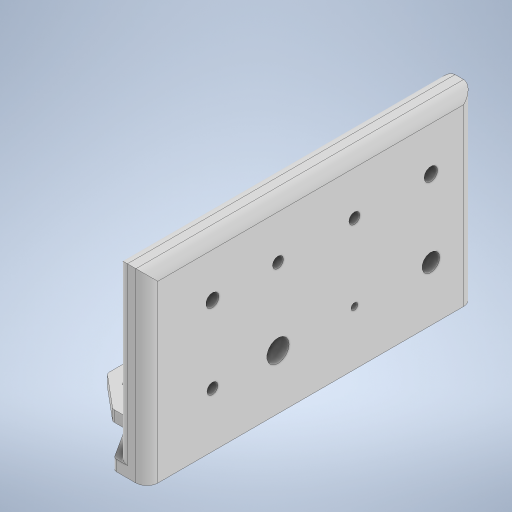
# Autodesk Inventor part: soporte_destornillador
Saved by Autodesk Inventor 2024 (Build 280153000, 153)
## iProperties
Created: 2023-06-27
Part Number: soporte_destornillador
Material: Generic
Document SubType Name: Modeling
Designer: LabTel_Admin
Density: 1 g/cm^3
Appearance: Default
Author: LabTel_Admin
Autodesk Inventor part; units mm, degrees
ref_plane "YZ Plane" through (0, 0, 0) normal (1, 0, 0) x (0, 1, 0)
ref_plane "XZ Plane" through (0, 0, 0) normal (0, 1, 0) x (-1, 0, 0)
ref_plane "XY Plane" through (0, 0, 0) normal (0, 0, 1) x (1, 0, 0)
sketch "Sketch2" plane through (0, 0, 0) normal (0, 1, 0) x (-1, 0, 0)
  line L0 (15.1065, 40) -> (17.4159, 44)
  line L1 (17.4159, 44) -> (22.0347, 44)
  line L2 (22.0347, 44) -> (24.3441, 40)
  line L3 (24.3441, 40) -> (22.0347, 36)
  line L4 (22.0347, 36) -> (17.4159, 36)
  line L5 (17.4159, 36) -> (15.1065, 40)
  circle A0 centre (19.7253, 40) radius 2.55
  line L6 (-20.2747, -75) -> (-20.2747, 75)
  line L7 (0, 0) -> (41.3759, 0) construction
  line L8 (15.1065, -40) -> (17.4159, -44)
  line L9 (17.4159, -44) -> (22.0347, -44)
  line L10 (22.0347, -44) -> (24.3441, -40)
  line L11 (24.3441, -40) -> (22.0347, -36)
  line L12 (22.0347, -36) -> (17.4159, -36)
  line L13 (17.4159, -36) -> (15.1065, -40)
  circle A1 centre (19.7253, -40) radius 2.55
  line L14 (29.108, 43.6367) -> (15.0592, 55.425)
  line L15 (29.8225, 43.0372) -> (48.1619, 43.0372) construction
  line L16 (13.7736, 55.8929) -> (8.0923, 55.8929)
  line L17 (29.108, -43.6367) -> (15.0592, -55.425)
  line L18 (13.7736, -55.8929) -> (8.0923, -55.8929)
  line L19 (29.8225, 42.1046) -> (29.8225, -42.1046)
  line L20 (-20.2747, 75) -> (-6.367, 75)
  line L21 (-4.6843, 74.081) -> (6.4096, 56.812)
  arc A2 (-4.6843, 74.081) -> (-6.367, 75) centre (-6.367, 73) ccw
  arc A3 (6.4096, 56.812) -> (8.0923, 55.8929) centre (8.0923, 57.8929) ccw
  arc A4 (15.0592, 55.425) -> (13.7736, 55.8929) centre (13.7736, 53.8929) ccw
  arc A5 (29.8225, 42.1046) -> (29.108, 43.6367) centre (27.8225, 42.1046) ccw
  arc A6 (29.108, -43.6367) -> (29.8225, -42.1046) centre (27.8225, -42.1046) ccw
  arc A7 (13.7736, -55.8929) -> (15.0592, -55.425) centre (13.7736, -53.8929) ccw
  line L22 (-20.2747, -75) -> (-6.367, -75)
  line L23 (-4.6843, -74.081) -> (6.4096, -56.812)
  arc A8 (-6.367, -75) -> (-4.6843, -74.081) centre (-6.367, -73) ccw
  arc A9 (8.0923, -55.8929) -> (6.4096, -56.812) centre (8.0923, -57.8929) ccw
  point P0 (19.7253, 36)
  point P1 (19.7253, 44)
  point P2 (23.1894, 42)
  point P3 (19.7253, -36)
  point P4 (19.7253, -44)
  point P5 (23.1894, -42)
  point P6 (14.5016, 55.8929)
  point P7 (7, 55.8929)
  point P8 (29.8225, -43.0372)
  point P9 (14.5016, -55.8929)
  point P10 (7, -55.8929)
  point P11 (-5.2747, 75)
  point P12 (-5.2747, -75)
  dimension "d18" = 8
  dimension "d19" = 5.1
  dimension "d60" = 150
  dimension "d62" = 40
  dimension "d63" = 40
  dimension "d64" = 20
  dimension "d65" = 140
  dimension "d66" = 75
  dimension "d67" = 15
  dimension "d68" = 2
  dimension "d69" = 15
  dimension "d70" = 2
  constraints: 48 end point, 16 point on circle, 16 point on line, 16 tangent, 14 symmetric about line, 10 centre point, 6 equal radius, 4 horizontal, 3 coincident, 3 midpoint, 2 vertical, 1 equal length, 14 other
  measures "d18" distance of point (19.725, 36) point (19.725, 44)
  measures "d19" diameter of A0
  measures "d60" distance of L6.start L6.end
  measures "d62" distance from line of L7 point (19.725, 40)
  measures "d63" distance from line of L6 point (19.725, 40)
  measures "d64" distance of L15.start point (14.502, 55.893)
  measures "d65" angle of L15 L14
  measures "d66" distance from line of L7 L6.end
  measures "d67" distance of L6.end point (-5.275, 75)
  measures "d68" radius of A2
  measures "d69" distance of L6.start point (-5.275, -75)
  measures "d70" radius of A8
extrude "Extrusion11" add sketch "Sketch2" along normal blind 5 contours L6 L20 A2 L21 A3 L16 A4 L14 A5 L19 A6 L17 A7 L18 A9 L23 A8 L22
extrude "Extrusion12" add sketch "Sketch2" along normal blind 3 contours L0 L1 L2 L3 L4 L5 | L13 L12 L11 L10 L9 L8
sketch "Sketch5" plane through (0, 5, 0) normal (0, 1, 0) x (1, 0, 0)
  line L0 (6.367, -75) -> (20.2747, -75) projected
  line L1 (20.2747, -75) -> (20.2747, 75) projected
  line L2 (6.367, -75) -> (20.2747, -75)
  line L3 (20.2747, -75) -> (20.2747, 75)
  line L4 (20.2747, 75) -> (6.367, 75)
  line L5 (6.367, 75) -> (6.367, -75)
  point P0 (0, 0)
  constraints: 8 end point, 2 parallel, 1 horizontal, 1 perpendicular
extrude "Extrusion13" add sketch "Sketch5" along normal blind 80
fillet "Fillet1" radius 5 6 edges at (6.367, 45, 75) (20.2747, 42.5, 75) (6.367, 85, 0) (20.2747, 85, 0) (6.367, 45, -75) (20.2747, 42.5, -75)
sketch "Sketch6" plane through (6.367, 5, -70) normal (-1, 0, 0) x (0, 0, 1)
  line L0 (0, 0) -> (0, 75) projected
  line L1 (140, 75) -> (140, 0) construction
  line L2 (140, 0) -> (140, 75)
  line L3 (145, 80) -> (145, -5) projected
  line L4 (0, 75) -> (140, 75) projected
  line L5 (115, 75) -> (115, 0) construction
  line L6 (85, 75) -> (85, 0) construction
  line L7 (50, 75) -> (50, 0) construction
  line L8 (15, 75) -> (15, 0) construction
  line L9 (140, -5) -> (140, 75) projected
  circle A0 centre (115, 55) radius 3
  circle A1 centre (85, 55) radius 2.5
  circle A2 centre (50, 55) radius 2.5
  circle A3 centre (15, 55) radius 3.075
  circle A4 centre (115, 55) radius 5.7
  circle A5 centre (85, 55) radius 5
  circle A6 centre (115, 20) radius 2.5
  circle A7 centre (85, 20) radius 5.1
  circle A8 centre (50, 20) radius 1.55
  circle A9 centre (15, 20) radius 4.05
  line L10 (140, 20) -> (0, 20) construction
  line L11 (140, 55) -> (0, 55) construction
  point P0 (70, -5)
  dimension "d79" = 75
  dimension "d82" = 25
  dimension "d83" = 30
  dimension "d84" = 35
  dimension "d85" = 35
  dimension "d86" = 20
  dimension "d87" = 6
  dimension "d88" = 11.4
  dimension "d89" = 5
  dimension "d90" = 10
  dimension "d91" = 5
  dimension "d92" = 6.15
  dimension "d93" = 20
  dimension "d94" = 5
  dimension "d95" = 10.2
  dimension "d96" = 3.1
  dimension "d97" = 8.1
  constraints: 24 point on line, 14 end point, 10 centre point, 4 vertical, 2 coincident, 2 perpendicular, 1 parallel
  measures "d79" distance of L1.start L1.end
  measures "d82" distance from line of L1 L5.start
  measures "d83" distance of L6.start L5.start
  measures "d84" distance of L7.start L6.start
  measures "d85" distance of L8.start L7.start
  measures "d86" distance of L1.start L11.start
  measures "d87" diameter of A0
  measures "d88" diameter of A4
  measures "d89" diameter of A1
  measures "d90" diameter of A5
  measures "d91" diameter of A2
  measures "d92" diameter of A3
  measures "d93" distance of L1.end L10.start
  measures "d94" diameter of A6
  measures "d95" diameter of A7
  measures "d96" diameter of A8
  measures "d97" diameter of A9
extrude "Extrusion14" cut sketch "Sketch6" against normal through all contours A0 | A1 | A2 | A3 | A6 | A7 | A8 | A9
extrude "Extrusion15" cut sketch "Sketch6" against normal blind 6 contours A4
extrude "Extrusion16" cut sketch "Sketch6" against normal blind 3.75 contours A5
body "Solid2"
